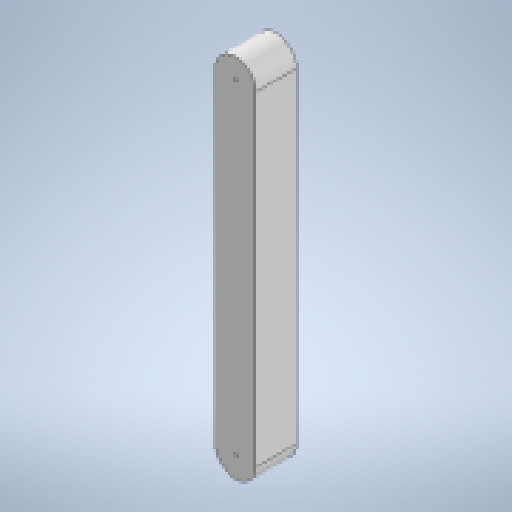
# Autodesk Inventor part: link2
Saved by Autodesk Inventor 2025.4 (Build 294407000, 407)
## iProperties
Created: 2026-03-19
Part Number: link2
Material: Generic
Document SubType Name: Modeling
Designer: dawid
Density: 1 g/cm^3
Appearance: Default
Author: dawid
Autodesk Inventor part; units mm, degrees
ref_plane "YZ Plane" through (0, 0, 0) normal (1, 0, 0) x (0, 1, 0)
ref_plane "XZ Plane" through (0, 0, 0) normal (0, 1, 0) x (-1, 0, 0)
ref_plane "XY Plane" through (0, 0, 0) normal (0, 0, 1) x (1, 0, 0)
sketch "Sketch1" plane through (0, 0, 0) normal (0, 0, 1) x (1, 0, 0)
  circle A0 centre (0, -75) radius 5
  arc A1 (-75, -75) -> (75, -75) centre (0, -75) ccw
  line L0 (-75, -75) -> (-75, 1225)
  arc A2 (75, 1225) -> (-75, 1225) centre (0, 1225) ccw
  circle A3 centre (0, 1225) radius 5
  line L1 (75, 1225) -> (75, -75)
  point P0 (0, 0)
  dimension "d0" = 10
  dimension "d1" = 150
  dimension "d3" = 1300
  dimension "d4" = 75
  constraints: 4 centre point, 4 end point, 4 point on circle, 4 tangent, 2 coincident, 2 equal radius, 1 vertical, 1 vertical alignment
  measures "d0" diameter of A0
  measures "d1" diameter of A1
  measures "d3" distance of L1.start L1.end
  measures "d4" distance of point (0, 0) A0.centre
extrude "Extrusion1" add sketch "Sketch1" along normal blind 150
equation "\"d4\" = 0.5 * d1"
body "Solid1"
